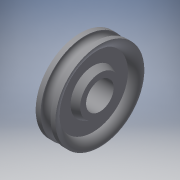
# Autodesk Inventor part: pulley
Saved by Autodesk Inventor 2019 (Build 230136000, 136)
## iProperties
Created: 2018-11-24
Part Number: pulley
Material: Generic
Document SubType Name: Modeling
Designer: Radek
Density: 1 g/cm^3
Appearance: Default
Author: Radek
Autodesk Inventor part; units mm, degrees
ref_plane "YZ Plane" through (0, 0, 0) normal (1, 0, 0) x (0, 1, 0)
ref_plane "XZ Plane" through (0, 0, 0) normal (0, 1, 0) x (-1, 0, 0)
ref_plane "XY Plane" through (0, 0, 0) normal (0, 0, 1) x (1, 0, 0)
sketch "Náčrt1" plane through (0, 0, 0) normal (0, 1, 0) x (-1, 0, 0)
  line L0 (10, -14) -> (0, -14)
  line L1 (10, -14) -> (10, -20)
  line L2 (10, -20) -> (3, -22.687)
  line L3 (3, -22.687) -> (3, -35.4606)
  line L4 (0, 0) -> (-43.8955, 0)
  arc A0 (10, -45) -> (3, -35.4606) centre (0, -45) ccw
  line L5 (0, 0) -> (0, -73.1539)
  line L6 (10, -45) -> (5, -45)
  arc A1 (5, -45) -> (0, -40) centre (0, -45) ccw
  line L7 (24.648, -45) -> (-37.389, -45)
  line L8 (10, -45) -> (10, -56.6969)
  line L9 (-10, -14) -> (0, -14)
  line L10 (-10, -14) -> (-10, -20)
  line L11 (-10, -20) -> (-3, -22.687)
  line L12 (-3, -22.687) -> (-3, -35.4606)
  arc A2 (-3, -35.4606) -> (-10, -45) centre (0, -45) ccw
  line L13 (-10, -45) -> (-5, -45)
  arc A3 (0, -40) -> (-5, -45) centre (0, -45) ccw
  point P0 (0, -53)
  dimension "d1" = 111
  dimension "d3" = 28
  dimension "d63" = 10
  dimension "d64" = 5
  dimension "d65" = 6
  dimension "d67" = 80
  dimension "d68" = 6
  constraints: 28 end point, 8 point on circle, 6 symmetric about line, 5 point on line, 4 centre point, 4 horizontal, 3 vertical, 2 coincident, 2 collinear, 1 parallel, 2 other
  measures "d1" angle of L3 L2
  measures "d3" diameter of L0 L4
  measures "d63" radius of A0
  measures "d64" radius of A1
  measures "d65" diameter of L3 L5
  measures "d67" diameter of A1.end L4
  measures "d68" distance of L0.start L1.end
revolve "Rotace1" add sketch "Náčrt1" angle 360 about axis through (0, 0, 0) along (1, 0, 0) contours L1 L2 L3 A0 L6 A1 L5 L0 | L5 A3 L7 A2 L12 L11 L10 L9
